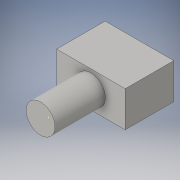
# Autodesk Inventor part: MCDAVE_SWITCH
Saved by Autodesk Inventor 2016 (Build 200138000, 138)
## iProperties
Created: 2017-09-08
Part Number: MCDAVE_SWITCH
Material: Generic
Document SubType Name: Modeling
Designer: student
Density: 1 g/cm^3
Appearance: Default
Author: student
Autodesk Inventor part; units mm, degrees
ref_plane "YZ Plane" through (0, 0, 0) normal (1, 0, 0) x (0, 1, 0)
ref_plane "XZ Plane" through (0, 0, 0) normal (0, 1, 0) x (-1, 0, 0)
ref_plane "XY Plane" through (0, 0, 0) normal (0, 0, 1) x (1, 0, 0)
sketch "Sketch1" plane through (0, 0, 0) normal (0, 0, 1) x (1, 0, 0)
  line L0 (-7.9265, 2.4178) -> (4.9259, 2.4178)
  line L1 (4.9259, 2.4178) -> (4.9259, -4.2624)
  line L2 (4.9259, -4.2624) -> (-7.9265, -4.2624)
  line L3 (-7.9265, -4.2624) -> (-7.9265, 2.4178)
  point P0 (0, 0)
  dimension "d0" = 6.6802
  dimension "d1" = 12.8524
  constraints: 8 end point, 2 parallel, 1 horizontal, 1 perpendicular
  measures "d0" distance of L2.end L0.start
  measures "d1" distance of L0.start L0.end
extrude "Extrusion1" add sketch "Sketch1" along normal blind 9.0932
sketch "Sketch2" plane through (0, 0, 9.0932) normal (0, 0, 1) x (1, 0, 0)
  line L0 (-7.9265, 2.4178) -> (-7.9265, -4.2624) projected
  line L1 (-7.9265, -0.9223) -> (4.9259, -0.9223)
  line L2 (4.9259, -4.2624) -> (4.9259, 2.4178) projected
  circle A0 centre (-1.5003, -0.9223) radius 2.7051
  point P0 (0, 0)
  dimension "d4" = 5.4102
  constraints: 3 midpoint, 2 end point, 1 centre point
  measures "d4" diameter of A0
extrude "Extrusion2" add sketch "Sketch2" along normal blind 9.4488
sketch "Sketch3" plane through (-1.5003, -0.9223, 18.542) normal (0, 0, 1) x (1, 0, 0)
  point P0 (1.5003, 0.9223)
body "Solid1"
